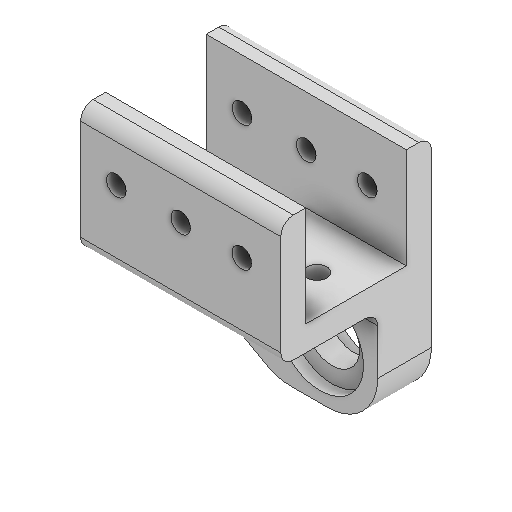
# Autodesk Inventor part: swingarmBase
Saved by Autodesk Inventor 2025 (Build 290162000, 162)
## iProperties
Created: 2024-10-14
Part Number: swingarmBase
Material: Generic
Document SubType Name: Modeling
Designer: derm
Density: 1 g/cm^3
Appearance: Default
Author: derm
Autodesk Inventor part; units mm, degrees
ref_plane "YZ Plane" through (0, 0, 0) normal (1, 0, 0) x (0, 1, 0)
ref_plane "XZ Plane" through (0, 0, 0) normal (0, 1, 0) x (-1, 0, 0)
ref_plane "XY Plane" through (0, 0, 0) normal (0, 0, 1) x (1, 0, 0)
sketch "Sketch1" plane through (0, 0, 0) normal (1, 0, 0) x (0, 1, 0)
  line L0 (-12.7635, 12.7635) -> (12.7635, 12.7635)
  line L1 (12.7635, 12.7635) -> (12.7635, -12.7635)
  line L2 (12.7635, -12.7635) -> (-12.7635, -12.7635)
  line L3 (-12.7635, -12.7635) -> (-12.7635, 12.7635)
  line L4 (-12.7635, 12.7635) -> (12.7635, -12.7635) construction
  line L5 (12.7635, 12.7635) -> (-12.7635, -12.7635) construction
  line L6 (19.1135, 19.1135) -> (-19.1135, 19.1135)
  line L7 (-19.1135, 19.1135) -> (-19.1135, -19.1135)
  line L8 (-19.1135, -19.1135) -> (19.1135, -19.1135)
  line L9 (19.1135, -19.1135) -> (19.1135, 19.1135)
  line L10 (12.7635, 19.1135) -> (12.7635, -19.1135)
  line L11 (-19.1135, -5.4793) -> (-46.5737, -5.4793)
  line L12 (-46.5737, -5.4793) -> (-46.5737, -19.1135)
  line L13 (-46.5737, -19.1135) -> (-19.1135, -19.1135)
  line L14 (-19.1135, -19.1135) -> (-19.1135, -5.4793)
  point P0 (0, 0)
  point P1 (12.7635, 12.7635)
  dimension "d1" = 25.527
  dimension "d2" = 6.35
  constraints: 30 end point, 6 parallel, 4 point on line, 3 perpendicular, 2 horizontal, 2 midpoint, 3 other
  measures "d1" distance of L1.end L2.end
  measures "d2" distance between parallel lines of L0 L6
extrude "Extrusion1" add sketch "Sketch1" along normal blind 50.8 contours L3 L2 L10 L8 L7 L6 L0 | L13 L12 L11 L7
sketch "Sketch2" plane through (0, -46.5737, -5.4793) normal (0, 0, 1) x (1, 0, 0)
  line L0 (0, 27.4602) -> (0, 0) projected
  line L1 (0, 0) -> (50.8, 0) projected
  line L2 (50.8, 27.4602) -> (50.8, 0) projected
  line L3 (0, 27.4602) -> (50.8, 27.4602) projected
  circle A0 centre (36.2123, 13.7301) radius 7
  point P0 (0, 46.5737)
  dimension "d5" = 14
  constraints: 1 centre point
  measures "d5" diameter of A0
extrude "Extrusion2" cut sketch "Sketch2" against normal through all contours A0
sketch "Sketch3" plane through (0, -46.5737, -19.1135) normal (0, 0, -1) x (-1, 0, 0)
  circle A0 centre (-36.2123, 13.7301) radius 7 projected
  circle A1 centre (-36.2123, 13.7301) radius 11
  point P0 (0, 46.5737)
  dimension "d8" = 22
  constraints: 1 centre point, 1 coincident
  measures "d8" diameter of A1
extrude "Extrusion3" cut sketch "Sketch3" against normal blind 5
sketch "Sketch4" plane through (0, -12.7635, 12.7635) normal (0, 1, 0) x (1, 0, 0)
  line L0 (0, 25.527) -> (0, 0) projected
  line L1 (0, 0) -> (50.8, 0) projected
  line L2 (50.8, 25.527) -> (50.8, 0) projected
  line L3 (0, 25.527) -> (50.8, 25.527) projected
  line L4 (0, 12.7635) -> (50.8, 12.7635) construction
  circle A0 centre (9.0739, 12.7635) radius 2.5
  circle A1 centre (25.4, 12.7635) radius 2.5
  circle A2 centre (40.9031, 12.7635) radius 2.5
  dimension "d11" = 5
  dimension "d12" = 5
  dimension "d13" = 5
  constraints: 3 centre point, 2 end point, 2 midpoint, 2 point on line
  measures "d11" diameter of A1
  measures "d12" diameter of A0
  measures "d13" diameter of A2
extrude "Extrusion4" cut sketch "Sketch4" against normal through all contours A0 | A1 | A2
sketch "Sketch5" plane through (0, -12.7635, 12.7635) normal (0, 0, -1) x (-1, 0, 0)
  line L0 (-43.4031, 0) -> (-38.4031, 0) projected
  line L1 (-27.9, 0) -> (-22.9, 0) projected
  line L2 (-11.5739, 0) -> (-6.5739, 0) projected
  line L3 (0, 0) -> (0, 25.527) projected
  line L4 (0, 25.527) -> (-50.8, 25.527) projected
  line L5 (-50.8, 0) -> (-50.8, 25.527) projected
  line L6 (0, 0) -> (-50.8, 0) projected
  circle A0 centre (-9.0739, 12.7635) radius 2.5
  circle A1 centre (-25.4, 12.7635) radius 2.5
  circle A2 centre (-40.9031, 12.7635) radius 2.5
  point P0 (0, 12.7635)
  dimension "d16" = 5
  constraints: 3 centre point, 2 equal radius
  measures "d16" diameter of A2
extrude "Extrusion5" cut sketch "Sketch5" along normal through all both and the other way through all contours A0 | A1 | A2
sketch "Sketch7" plane through (0, -46.5737, -5.4793) normal (0, 0, 1) x (1, 0, 0)
  circle A0 centre (36.2123, 13.7301) radius 7 projected
  circle A1 centre (36.2123, 13.7301) radius 11
  point P0 (0, 46.5737)
  dimension "d21" = 22
  constraints: 1 centre point, 1 coincident
  measures "d21" diameter of A1
extrude "Extrusion7" cut sketch "Sketch7" against normal blind 3
sketch "Sketch8" plane through (0, -46.5737, -5.4793) normal (0, 0, 1) x (1, 0, 0)
  line L0 (0, 27.4602) -> (0, 0) projected
  circle A0 centre (36.2123, 13.7301) radius 11 projected
  line L1 (0, 27.4602) -> (0, 0) projected
  line L2 (0, 0) -> (50.8, 0) projected
  line L3 (50.8, 27.4602) -> (50.8, 0) projected
  line L4 (0, 27.4602) -> (50.8, 27.4602) projected
  circle A1 centre (9.5855, 21.0501) radius 2.5
  line L5 (0, 0) -> (0, 59.3372) projected
  line L6 (0, 14.2925) -> (25.4, 0)
  point P0 (0, 46.5737)
  point P1 (0, 14.2925)
  dimension "d24" = 5
  constraints: 2 end point, 1 centre point, 1 midpoint, 1 point on line
  measures "d24" diameter of A1
extrude "Extrusion8" cut sketch "Sketch8" along normal through all both and the other way through all contours L6 L2 L0 | A1
fillet "Fillet1" radius 12.7 3 edges at (0, -32.2813, -12.2964) (50.8, -46.5737, -12.2964) (25.4, -46.5737, -12.2964)
sketch "Sketch9" plane through (0, -19.1135, -5.4793) normal (0, 0, 1) x (1, 0, 0)
  circle A0 centre (9.5855, -6.4101) radius 2.5 projected
  circle A1 centre (36.2123, -13.7301) radius 11 projected
  arc A2 (22.4998, -25.8283) -> (28.7278, -27.4602) centre (28.7278, -14.7602) ccw projected
  line L0 (28.7278, -27.4602) -> (38.1, -27.4602) projected
  arc A3 (38.1, -27.4602) -> (50.8, -14.7602) centre (38.1, -14.7602) ccw projected
  line L1 (50.8, 0) -> (50.8, -14.7602) projected
  line L2 (0, 0) -> (50.8, 0) projected
  line L3 (0, 0) -> (0, -5.7415) projected
  arc A4 (0, -5.7415) -> (6.472, -16.8095) centre (12.7, -5.7415) ccw projected
  line L4 (6.472, -16.8095) -> (22.4998, -25.8283) projected
  circle A5 centre (9.5855, -6.4101) radius 5.3589
  point P0 (0, 19.1135)
  constraints: 1 centre point, 1 coincident
extrude "Extrusion9" cut sketch "Sketch9" against normal blind 5 contours A5
fillet "Fillet2" radius 3.175 1 edges at (25.4, -19.1135, -5.4793)
fillet "Fillet3" radius 3.175 3 edges at (25.4, -19.1135, 19.1135) (25.4, 12.7635, 19.1135) (25.4, 12.7635, -19.1135)
body "Solid1"
